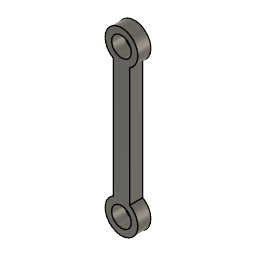
Spanner (Autodesk Fusion 360 design; units mm, degrees)
part number: 2026-03-10-20-56-15-167
Autodesk Fusion 360 part; units mm, degrees
sketch "Sketch1" plane through (0, 0, 0) normal (0, 0, 1) x (1, 0, 0)
sketch "Sketch2" plane through (0, 0, 0) normal (0, 1, 0) x (1, 0, 0)
  circle A0 centre (-0.2273, -83.6981) radius 3
  circle A1 centre (-0.2269, -38.6981) radius 3
  line L0 (-2.7272, -43.028) -> (-2.7272, -79.3679)
  line L1 (2.2731, -43.0282) -> (2.2731, -79.3682)
  arc A2 (-2.7272, -79.3679) -> (2.2731, -79.3682) centre (-0.2273, -83.6981) ccw
  arc A3 (2.2731, -43.0282) -> (-2.7272, -43.028) centre (-0.2269, -38.6981) ccw
  point P0 (-0.2269, -38.6981)
  dimension "d1" = 6
  dimension "d2" = 6
  dimension "d3" = 10
  dimension "d4" = 10
  dimension "d5" = 45
  dimension "d7" = 36.34
  constraint concentric A0 A2
  constraint concentric A1 A3
  constraint coincident P0 A1.centre
  constraint vertical L0
  constraint vertical L1
  measures "d1" diameter of A0
  measures "d2" diameter of A1
  measures "d3" diameter of A2
  measures "d4" diameter of A3
  measures "d5" distance of P0 A0.centre
  measures "d7" distance of L1.start L1.end
extrude "Extrude1" add sketch "Sketch2" along normal blind 4
